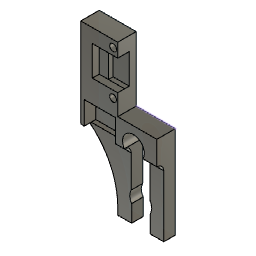
Y Stop-block (Autodesk Fusion 360 design; units mm, degrees)
Autodesk Fusion 360 part; units mm, degrees
sketch "Sketch1" plane through (0, 0, 0) normal (1, 0, 0) x (0, 1, 0) in component "Component"
  line L0 (0, 0) -> (1, 0)
  line L1 (1, 0) -> (1, 40)
  line L2 (1, 40) -> (0, 40)
  line L3 (0, 40) -> (0, 0)
  dimension "d3" = 1
  dimension "d4" = 40
  constraint horizontal L0
  constraint vertical L1
  constraint horizontal L2
  constraint vertical L3
  constraint coincident L0.start L3.end
  measures "d3" distance of L0.start L0.end
  measures "d4" distance of L0.start L2.end
extrude "Extrude1" add sketch "Sketch1" against normal blind 20 in component "Component"
sketch "Sketch2" plane through (0, 1, 0) normal (0, 1, 0) x (-1, 0, 0) in component "Component"
  line L0 (0, 40) -> (0, 0)
  line L1 (0, 0) -> (20, 0)
  line L2 (20, 0) -> (20, 40)
  line L3 (20, 40) -> (0, 40)
  line L4 (6.0137, 29.6802) -> (6.0137, 12.583)
  line L5 (14.1333, 29.3642) -> (14.1333, 12.3406)
  arc A0 (14.1333, 29.3642) -> (6.0137, 29.6802) centre (10.1692, 31.9811) ccw
  line L6 (5.8481, 7.6926) -> (5.8481, 0)
  line L7 (13.9529, 7.3662) -> (13.9529, 0)
  arc A1 (6.0137, 12.583) -> (5.8481, 7.6926) centre (10, 10) ccw
  arc A2 (13.9529, 7.3662) -> (14.1333, 12.3406) centre (10, 10) ccw
  point P0 (10, 10)
  dimension "d7" = 9.5
  dimension "d8" = 9.5
  constraint coincident P0 A1.centre
  constraint vertical L4
  constraint parallel L2 L5
  constraint coincident L1 L6.end
  constraint perpendicular L1 L6
  constraint coincident L7.start A1
  constraint coincident L1 L7.end
  constraint perpendicular L1 L7
  constraint concentric A1 A2
  measures "d7" diameter of A0
  measures "d8" diameter of A1
extrude "Extrude2" cut sketch "Sketch2" against normal up to surface (1 mm away) contours L1 L4 L5 A0 L6 L7 A1 A2 in component "Component"
extrude "Extrude3" add 1 faces at (-18.2048, 0, 17.0423) along direction (0, -1, 0) blind 4 in component "Component"
extrude "Extrude4" add 1 faces at (-20, -2.3333, 26.6667) along direction (-1, 0, 0) blind 13 in component "Component"
sketch "Sketch3" plane through (0, 0, 40) normal (0, 0, 1) x (-1, 0, 0)
  line L0 (0, 4) -> (0, -1)
  line L1 (0, -1) -> (33, -1)
  line L2 (33, -1) -> (33, 4)
  line L3 (33, 4) -> (0, 4)
  line L4 (33, -1) -> (17, -1)
  line L5 (17, -1) -> (17, 4)
  line L6 (17, 4) -> (33, 4)
  line L7 (33, 4) -> (33, -1)
  dimension "d16" = 16
  constraint horizontal L4
  constraint vertical L5
  constraint horizontal L6
  constraint vertical L7
  constraint coincident L1.end L2.start
  measures "d16" distance of L1.end L4.end
extrude "Extrude5" add sketch "Sketch3" along normal blind 28 contours L1 L2 L3 L4 L5 L6 L7 in component "Component"
sketch "Sketch4" plane through (0, -4, 0) normal (0, -1, 0) x (1, 0, 0)
  line L0 (-13.9529, 0) -> (-13.9529, 7.3662)
  arc A0 (-14.1333, 12.3406) -> (-13.9529, 7.3662) centre (-10, 10) ccw
  line L1 (-14.1333, 12.3406) -> (-14.1333, 29.3642)
  arc A1 (-6.0137, 29.6802) -> (-14.1333, 29.3642) centre (-10.1692, 31.9811) ccw
  line L2 (-6.0137, 29.6802) -> (-6.0137, 12.583)
  arc A2 (-5.8481, 7.6926) -> (-6.0137, 12.583) centre (-10, 10) ccw
  line L3 (-5.8481, 7.6926) -> (-5.8481, 0)
  line L4 (-5.8481, 0) -> (0, 0)
  line L5 (0, 0) -> (0, 40)
  line L6 (0, 40) -> (-17, 40)
  line L7 (-17, 40) -> (-17, 68)
  line L8 (-17, 68) -> (-33, 68)
  line L9 (-33, 68) -> (-33, 0)
  line L10 (-33, 0) -> (-13.9529, 0)
  line L11 (-20, 0) -> (-20, 20)
  line L12 (-20, 20) -> (-33, 29.3642)
  line L13 (-33, 0) -> (-20, 0)
  line L14 (-33, 29.3642) -> (-33, 0)
  constraint coincident L10 L11.start
  constraint perpendicular L10 L11
  constraint coincident L9 L12.end
  constraint coincident L9.end L10.start
extrude "Extrude6" cut sketch "Sketch4" against normal up to surface (5 mm away) contours L9 L10 L11 L12 L13 L14 in component "Component"
fillet "Fillet2" radius 32.5 1 edges at (-20, -1.5, 20) in component "Component"
sketch "Sketch5" plane through (0, 1, 0) normal (0, 1, 0) x (-1, 0, 0)
  line L0 (20, 0) -> (20, 3.3642)
  arc A0 (33, 29.3642) -> (20, 3.3642) centre (52.5, 3.3642) ccw
  line L1 (33, 29.3642) -> (33, 68)
  line L2 (33, 68) -> (17, 68)
  line L3 (17, 68) -> (17, 40)
  line L4 (0, 40) -> (0, 0)
  line L5 (0, 0) -> (5.8481, 0)
  line L6 (5.8481, 0) -> (5.8481, 7.6926)
  arc A1 (6.0137, 12.583) -> (5.8481, 7.6926) centre (10, 10) ccw
  line L7 (6.0137, 12.583) -> (6.0137, 29.6802)
  arc A2 (14.1333, 29.3642) -> (6.0137, 29.6802) centre (10.1692, 31.9811) ccw
  line L8 (14.1333, 29.3642) -> (14.1333, 12.3406)
  arc A3 (13.9529, 7.3662) -> (14.1333, 12.3406) centre (10, 10) ccw
  line L9 (13.9529, 7.3662) -> (13.9529, 0)
  line L10 (13.9529, 0) -> (20, 0)
  line L11 (17, 40) -> (0, 40)
sketch "Sketch6" plane through (0, -4, 0) normal (0, -1, 0) x (1, 0, 0)
  line L0 (-20, 3.3642) -> (-20, 0)
  line L1 (-20, 0) -> (-13.9529, 0)
  line L2 (-13.9529, 0) -> (-13.9529, 7.3662)
  arc A0 (-14.1333, 12.3406) -> (-13.9529, 7.3662) centre (-10, 10) ccw
  line L3 (-14.1333, 12.3406) -> (-14.1333, 29.3642)
  arc A1 (-6.0137, 29.6802) -> (-14.1333, 29.3642) centre (-10.1692, 31.9811) ccw
  line L4 (-6.0137, 29.6802) -> (-6.0137, 12.583)
  arc A2 (-5.8481, 7.6926) -> (-6.0137, 12.583) centre (-10, 10) ccw
  line L5 (-5.8481, 7.6926) -> (-5.8481, 0)
  line L6 (-5.8481, 0) -> (0, 0)
  line L7 (0, 0) -> (0, 40)
  line L8 (-17, 40) -> (-17, 68)
  line L9 (-17, 68) -> (-33, 68)
  line L10 (-33, 68) -> (-33, 29.3642)
  arc A3 (-20, 3.3642) -> (-33, 29.3642) centre (-52.5, 3.3642) ccw
  line L11 (-17, 68) -> (-33, 68)
  line L12 (-33, 68) -> (-33, 62)
  line L13 (-17, 62) -> (-17, 68)
  line L14 (-17, 62) -> (-24, 62)
  line L15 (-24, 62) -> (-24, 49)
  line L16 (-24, 49) -> (-17, 49)
  line L17 (-17, 49) -> (-17, 62)
  line L18 (0, 40) -> (-17, 40)
  line L19 (-24, 39.2) -> (-17, 39.2)
  line L20 (-17, 39.2) -> (-31.5, 39.2)
  line L21 (-31.5, 39.2) -> (-31.5, 29.2)
  line L22 (-31.5, 29.2) -> (-17, 29.2)
  line L23 (-17, 29.2) -> (-17, 39.2)
  dimension "d25" = 6
  dimension "d26" = 7
  dimension "d27" = 13
  dimension "d28" = 9.8
  dimension "d30" = 10
  constraint horizontal L11
  constraint vertical L12
  constraint vertical L13
  constraint coincident L8.end L9.start
  constraint horizontal L14
  constraint vertical L15
  constraint horizontal L16
  constraint vertical L17
  constraint horizontal L19
  constraint horizontal L20
  constraint vertical L21
  constraint horizontal L22
  constraint vertical L23
  measures "d25" distance of L8.end L13.start
  measures "d26" distance of L13.start L14.end
  measures "d27" distance of L13.start L16.end
  measures "d28" distance of L15.end L19.start
  measures "d30" distance of L19.end L22.end
extrude "Extrude7" cut sketch "Sketch6" against normal blind 2 contours L8 L14 L15 L16 L17 | L19 L20 L21 L22 L23 in component "Component"
sketch "Sketch7" plane through (0, -4, 0) normal (0, -1, 0) x (1, 0, 0)
  line L0 (-24, 62) -> (-17, 62)
  line L1 (-17, 62) -> (-17, 68)
  line L2 (-17, 68) -> (-33, 68)
  line L3 (-33, 68) -> (-33, 29.3642)
  arc A0 (-20, 3.3642) -> (-33, 29.3642) centre (-52.5, 3.3642) ccw
  line L4 (-20, 3.3642) -> (-20, 0)
  line L5 (-20, 0) -> (-13.9529, 0)
  line L6 (-13.9529, 0) -> (-13.9529, 7.3662)
  arc A1 (-14.1333, 12.3406) -> (-13.9529, 7.3662) centre (-10, 10) ccw
  line L7 (-14.1333, 12.3406) -> (-14.1333, 29.3642)
  arc A2 (-6.0137, 29.6802) -> (-14.1333, 29.3642) centre (-10.1692, 31.9811) ccw
  line L8 (-6.0137, 29.6802) -> (-6.0137, 12.583)
  arc A3 (-5.8481, 7.6926) -> (-6.0137, 12.583) centre (-10, 10) ccw
  line L9 (-5.8481, 7.6926) -> (-5.8481, 0)
  line L10 (-5.8481, 0) -> (0, 0)
  line L11 (0, 0) -> (0, 40)
  line L12 (0, 40) -> (-17, 40)
  line L13 (-17, 40) -> (-17, 49)
  line L14 (-17, 49) -> (-24, 49)
  line L15 (-24, 49) -> (-24, 62)
  line L16 (-31.5, 39.2) -> (-17, 39.2)
  line L17 (-17, 39.2) -> (-17, 29.2)
  line L18 (-17, 29.2) -> (-31.5, 29.2)
  line L19 (-31.5, 29.2) -> (-31.5, 39.2)
  line L20 (-24, 62) -> (-28, 62)
  line L21 (-28, 62) -> (-28, 49)
  line L22 (-28, 49) -> (-24, 49)
  line L23 (-24, 49) -> (-24, 62)
  line L24 (-33, 39.2) -> (-33, 68)
  line L25 (-17, 68) -> (-17, 62)
  line L26 (-28, 49) -> (-17, 49)
  line L27 (-17, 39.2) -> (-31.5, 39.2)
  line L28 (-31.5, 29.2) -> (-33, 29.3642)
  line L29 (0, 29.6802) -> (-6.0137, 29.6802)
  line L30 (-14.1333, 29.3642) -> (-17, 29.3642)
  dimension "d33" = 4
  constraint horizontal L20
  constraint vertical L21
  constraint horizontal L22
  constraint vertical L23
  constraint coincident L0.start L15.end
  constraint coincident L16.start L19.end
  constraint coincident L3 L24.start
  constraint coincident L2.end L3.start
  constraint coincident L1.end L2.start
  constraint coincident L0.end L1.start
  constraint coincident L13.end L14.start
  constraint coincident L16.end L17.start
  constraint coincident L18.end L19.start
  constraint coincident L3.end A0.end
  constraint coincident L11 L29.start
  constraint coincident A2.start L8.start
  constraint perpendicular L8 L29
  constraint coincident L7.end A2.end
  constraint coincident L17 L30.end
  constraint perpendicular L17 L30
  measures "d33" distance of L0.start L20.end
extrude "Extrude8" add sketch "Sketch7" along normal blind 3 contours L0 L1 L2 L3 A2 L11 L12 L13 L14 L16 L17 L19 L20 L21 L22 L24 L25 L26 L27 L28 L29 L30 in component "Component"
fillet "Fillet3" radius 3 2 edges at (-3.0068, -4, 29.6802) (-15.5667, -4, 29.3642) in component "Component"
extrude "Extrude9" add 6 faces at (-17, -5, 33.5326) (-17, -5, 38.0056) (-17, -4.6737, 29.2547) (-17, -2.6667, 31.3937) (-17, -3.3333, 36.8112) (-17, -4.5494, 28.6794) along direction (-1, 0, 0) blind 1 in component "Component"
sketch "Sketch8" plane through (0, -7, 0) normal (0, -1, 0) x (1, 0, 0)
  line L0 (0, 29.6802) -> (0, 40)
  line L1 (0, 40) -> (-17, 40)
  line L2 (-17, 40) -> (-17, 49)
  line L3 (-17, 49) -> (-28, 49)
  line L4 (-28, 49) -> (-28, 62)
  line L5 (-28, 62) -> (-17, 62)
  line L6 (-17, 62) -> (-17, 68)
  line L7 (-17, 68) -> (-33, 68)
  line L8 (-33, 68) -> (-33, 39.2)
  line L9 (-33, 39.2) -> (-33, 29.3642)
  line L10 (-33, 29.3642) -> (-31.5, 29.2)
  line L11 (-31.5, 29.2) -> (-31.5, 39.2)
  line L12 (-31.5, 39.2) -> (-18, 39.2)
  line L13 (-18, 39.2) -> (-18, 29.3642)
  line L14 (-18, 29.3642) -> (-14.1333, 29.3642)
  arc A0 (-6.0137, 29.6802) -> (-14.1333, 29.3642) centre (-10.1692, 31.9811) ccw
  line L15 (-6.0137, 29.6802) -> (0, 29.6802)
  circle A1 centre (-19, 65) radius 1.5
  circle A2 centre (-19, 46) radius 1.5
  dimension "d42" = 3
  dimension "d44" = 3
  measures "d42" diameter of A1
  measures "d44" diameter of A2
extrude "Extrude10" cut sketch "Sketch8" against normal up to surface (8 mm away) contours A1 | A2 in component "Component"
fillet "Fillet4" radius 0.5 tangency weight 0.94957 1 edges at (-32.25, -4, 29.2821) in component "Component"
component "Component" placed x (1, 0, 0) y (0, 1, 0) z (0, 0, 1) at (0, 0, 0)
